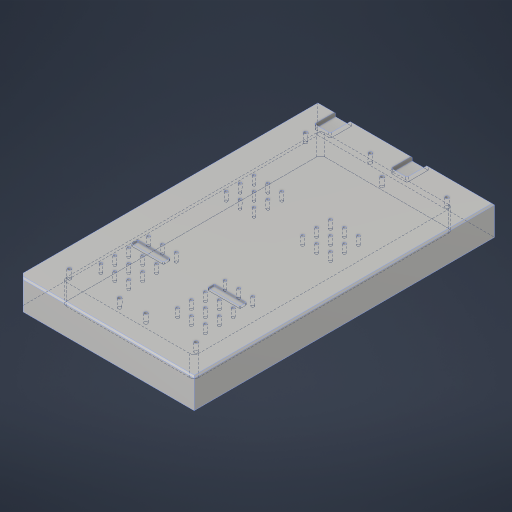
# Autodesk Inventor part: Assembly Plate
Saved by Autodesk Inventor 2024 (Build 280153000, 153)
## iProperties
Created: 2021-01-11
Part Number: Assembly Plate
Material: Aluminum 6061
Document SubType Name: Modeling
Designer: caleb
Density: 2.7 g/cm^3
Appearance: Aluminum - Flat
Author: caleb
Autodesk Inventor part; units mm, degrees
ref_plane "YZ Plane" through (0, 0, 0) normal (1, 0, 0) x (0, 1, 0)
ref_plane "XZ Plane" through (0, 0, 0) normal (0, 1, 0) x (-1, 0, 0)
ref_plane "XY Plane" through (0, 0, 0) normal (0, 0, 1) x (1, 0, 0)
sketch "Sketch1" plane through (0, 0, 0) normal (0, 1, 0) x (-1, 0, 0)
  line L0 (-63.5, 107.95) -> (63.5, 107.95)
  line L1 (63.5, 107.95) -> (63.5, -107.95)
  line L2 (63.5, -107.95) -> (-63.5, -107.95)
  line L3 (-63.5, -107.95) -> (-63.5, 107.95)
  line L4 (-63.5, 107.95) -> (63.5, -107.95) construction
  line L5 (63.5, 107.95) -> (-63.5, -107.95) construction
  point P0 (0, 0)
  dimension "d0" = 127
  dimension "d1" = 215.9
  constraints: 12 end point, 2 midpoint, 2 parallel, 1 horizontal, 1 perpendicular
  measures "d0" distance of L1.end L2.end
  measures "d1" distance of L0.end L1.end
extrude "Extrusion1" add sketch "Sketch1" along normal blind 21.14
sketch "Sketch9" plane through (0, 21.14, 0) normal (0, 1, 0) x (1, 0, 0)
  line L0 (-63.5, 107.95) -> (-63.5, -107.95) projected
  line L1 (-63.5, -107.95) -> (63.5, -107.95) projected
  point P0 (0, 0)
  point P1 (-48.5, -85.65)
  point P2 (-12.4, -85.65)
  point P3 (-48.5, 84.134)
  point P4 (-12.4, 94.65)
  point P5 (42.6, 94.65)
  point P6 (6.5, 84.134)
  point P7 (42.6, -85.65)
  point P8 (6.5, -85.65)
  dimension "d126" = 36.1
  dimension "d127" = 169.784
  dimension "d128" = 180.3
  dimension "d129" = 15
  dimension "d130" = 22.3
  dimension "d164" = 55
  constraints: 2 vertical alignment, 1 horizontal, 1 horizontal alignment, 4 other
  measures "d126" distance of point (-12.4, -85.65) point (-48.5, -85.65)
  measures "d127" distance of point (-48.5, 84.134) point (-48.5, -85.65)
  measures "d128" distance of point (-12.4, 94.65) point (-12.4, -85.65)
  measures "d129" distance from line of L0 point (-48.5, -85.65)
  measures "d130" vertical distance of L0.end point (-48.5, -85.65)
  measures "d164" distance of point (-12.4, 94.65) point (42.6, 94.65)
hole "Hole2" at (-48.5, 21.14, 85.65) at (-12.4, 21.14, 85.65) at (-48.5, 21.14, -84.134) at (-12.4, 21.14, -94.65) at (6.5, 21.14, 85.65) at (42.6, 21.14, 85.65) at (6.5, 21.14, -84.134) at (42.6, 21.14, -94.65) direction (0, -1, 0) diameter 2.5 end through all
sketch "Sketch10" plane through (0, 21.14, 0) normal (0, 1, 0) x (1, 0, 0)
  line L0 (-41.5, -47.65) -> (-19.4, -47.65)
  line L1 (-18.9, -47.15) -> (-18.9, -43.45)
  line L2 (-19.4, -42.95) -> (-41.5, -42.95)
  line L3 (-42, -43.45) -> (-42, -47.15)
  line L4 (-63.5, -107.95) -> (63.5, -107.95) projected
  line L5 (-63.5, 107.95) -> (-63.5, -107.95) projected
  arc A0 (-42, -47.15) -> (-41.5, -47.65) centre (-41.5, -47.15) ccw
  arc A1 (-41.5, -42.95) -> (-42, -43.45) centre (-41.5, -43.45) ccw
  arc A2 (-18.9, -43.45) -> (-19.4, -42.95) centre (-19.4, -43.45) ccw
  arc A3 (-19.4, -47.65) -> (-18.9, -47.15) centre (-19.4, -47.15) ccw
  arc A4 (13.5, -42.95) -> (13, -43.45) centre (13.5, -43.45) ccw
  arc A5 (36.1, -43.45) -> (35.6, -42.95) centre (35.6, -43.45) ccw
  line L6 (13, -43.45) -> (13, -47.15)
  line L7 (36.1, -47.15) -> (36.1, -43.45)
  line L8 (13.5, -47.65) -> (35.6, -47.65)
  arc A6 (13, -47.15) -> (13.5, -47.65) centre (13.5, -47.15) ccw
  arc A7 (35.6, -47.65) -> (36.1, -47.15) centre (35.6, -47.15) ccw
  line L9 (35.6, -42.95) -> (13.5, -42.95)
  point P0 (0, 0)
  point P1 (-42, -47.65)
  point P2 (-18.9, -42.95)
  point P3 (-18.9, -47.65)
  point P4 (-42, -42.95)
  point P5 (13, -47.65)
  point P6 (13, -42.95)
  point P7 (36.1, -42.95)
  point P8 (36.1, -47.65)
  dimension "d140" = 60.3
  dimension "d141" = 65
  dimension "d142" = 21.5
  dimension "d143" = 23.1
  dimension "d144" = 0.5
  dimension "d171" = 55
  constraints: 16 end point, 16 point on circle, 16 point on line, 8 centre point, 8 tangent, 3 equal radius, 2 horizontal, 2 parallel, 1 perpendicular, 24 other
  measures "d140" distance between parallel lines of L4 L0
  measures "d141" distance between parallel lines of L4 L2
  measures "d142" distance between parallel lines of L5 L3
  measures "d143" distance between parallel lines of L1 L3
  measures "d144" radius of A0
  measures "d171" distance of L3.start L6.start
extrude "Extrusion8" cut sketch "Sketch10" against normal blind 1.5
sketch "Sketch11" plane through (0, 21.14, 0) normal (0, 1, 0) x (1, 0, 0)
  line L0 (63.5, 107.95) -> (-63.5, 107.95) projected
  line L1 (-50.7, 107.95) -> (-39.2, 107.95)
  line L2 (-39.2, 107.95) -> (-39.2, 93.65)
  line L3 (-40.2, 92.65) -> (-49.7, 92.65)
  line L4 (-50.7, 93.65) -> (-50.7, 107.95)
  line L5 (-63.5, 107.95) -> (-63.5, -107.95) projected
  arc A0 (-50.7, 93.65) -> (-49.7, 92.65) centre (-49.7, 93.65) ccw
  arc A1 (-40.2, 92.65) -> (-39.2, 93.65) centre (-40.2, 93.65) ccw
  line L6 (4.3, 107.95) -> (15.8, 107.95)
  line L7 (15.8, 107.95) -> (15.8, 93.65)
  line L8 (14.8, 92.65) -> (5.3, 92.65)
  line L9 (4.3, 93.65) -> (4.3, 107.95)
  arc A2 (4.3, 93.65) -> (5.3, 92.65) centre (5.3, 93.65) ccw
  arc A3 (14.8, 92.65) -> (15.8, 93.65) centre (14.8, 93.65) ccw
  point P0 (0, 0)
  point P1 (-39.2, 92.65)
  point P2 (-50.7, 92.65)
  point P3 (-39.2, 100.8)
  point P4 (15.8, 92.65)
  point P5 (4.3, 92.65)
  point P6 (15.8, 100.8)
  dimension "d145" = 12.8
  dimension "d146" = 24.3
  dimension "d147" = 15.3
  dimension "d150" = 1
  dimension "d178" = 55
  constraints: 16 end point, 9 point on line, 8 point on circle, 4 centre point, 4 tangent, 2 horizontal, 2 parallel, 1 equal radius, 1 midpoint, 1 perpendicular, 17 other
  measures "d145" distance between parallel lines of L5 L4
  measures "d146" distance from line of point (-39.2, 100.8) L5
  measures "d147" distance between parallel lines of L0 L3
  measures "d150" radius of A0
  measures "d178" distance of L1.start L6.start
extrude "Extrusion9" cut sketch "Sketch11" against normal blind 3.25
chamfer "Chamfer2" distance 1 angle 45 6 edges at (63.5, 21.14, 0) (-57.1, 21.14, -107.95) (-17.45, 21.14, -107.95) (39.65, 21.14, -107.95) (-63.5, 21.14, 0) (0, 21.14, 107.95)
sketch "Sketch12" plane through (0, 0, 0) normal (0, -1, 0) x (1, 0, 0)
  line L0 (-47.5, -96.95) -> (41.5, -96.95)
  line L1 (44.5, -93.95) -> (44.5, 85.95)
  line L2 (41.5, 88.95) -> (-47.5, 88.95)
  line L3 (-50.5, 85.95) -> (-50.5, -93.95)
  line L4 (63.5, -107.95) -> (63.5, 107.95) projected
  line L5 (63.5, 107.95) -> (-63.5, 107.95) projected
  arc A0 (44.5, 85.95) -> (41.5, 88.95) centre (41.5, 85.95) ccw
  arc A1 (-47.5, 88.95) -> (-50.5, 85.95) centre (-47.5, 85.95) ccw
  arc A2 (-50.5, -93.95) -> (-47.5, -96.95) centre (-47.5, -93.95) ccw
  arc A3 (41.5, -96.95) -> (44.5, -93.95) centre (41.5, -93.95) ccw
  line L6 (-63.5, -107.95) -> (-63.5, 107.95) projected
  line L7 (63.5, -107.95) -> (15.8, -107.95) projected
  point P0 (0, 0)
  point P1 (63.5, 103.95)
  point P2 (59.5, 107.95)
  point P3 (-39.2, -107.95)
  dimension "d151" = 19
  dimension "d152" = 19
  dimension "d153" = 3
  dimension "d160" = 13
  dimension "d161" = 11
  constraints: 8 end point, 8 point on circle, 8 tangent, 4 centre point, 3 equal radius, 2 parallel, 1 horizontal, 1 perpendicular
  measures "d151" distance between parallel lines of L4 L1
  measures "d152" distance between parallel lines of L5 L2
  measures "d153" radius of A0
  measures "d160" distance between parallel lines of L6 L3
  measures "d161" distance between parallel lines of L7 L0
extrude "Extrusion10" cut sketch "Sketch12" against normal blind 15
chamfer "Chamfer4" distance 4 angle 45 1 edges at (-63.5, 10.07, 107.95)
sketch "Sketch13" plane through (0, 21.14, 0) normal (0, 1, 0) x (1, 0, 0)
  line L0 (-63.5, 107.95) -> (-63.5, -103.95) projected
  line L1 (-59.5, -107.95) -> (63.5, -107.95) projected
  point P0 (0, 0)
  point P1 (-40.5, -70.95)
  point P2 (-40.5, -60.95)
  point P3 (-40.5, -50.95)
  point P4 (-30.5, -70.95)
  point P5 (-30.5, -60.95)
  point P6 (-30.5, -50.95)
  point P7 (-20.5, -70.95)
  point P8 (-20.5, -60.95)
  point P9 (-20.5, -50.95)
  point P10 (-20.5, 39.05)
  point P11 (-20.5, 29.05)
  point P12 (-20.5, 19.05)
  point P13 (-30.5, 39.05)
  point P14 (-30.5, 29.05)
  point P15 (-30.5, 19.05)
  point P16 (-40.5, 39.05)
  point P17 (-40.5, 29.05)
  point P18 (-40.5, 19.05)
  point P19 (34.5, -50.95)
  point P20 (34.5, -60.95)
  point P21 (34.5, -70.95)
  point P22 (24.5, -50.95)
  point P23 (24.5, -60.95)
  point P24 (24.5, -70.95)
  point P25 (14.5, -50.95)
  point P26 (14.5, -60.95)
  point P27 (14.5, -70.95)
  point P28 (34.5, 39.05)
  point P29 (34.5, 29.05)
  point P30 (34.5, 19.05)
  point P31 (24.5, 39.05)
  point P32 (24.5, 29.05)
  point P33 (24.5, 19.05)
  point P34 (14.5, 39.05)
  point P35 (14.5, 29.05)
  point P36 (14.5, 19.05)
  point P37 (-40.5, -36.8096)
  point P38 (-30.5, -36.8096)
  point P39 (-20.5, -36.8096)
  point P40 (14.5, -36.8096)
  point P41 (24.5, -36.8096)
  point P42 (34.5, -36.8096)
  dimension "d185" = 10
  dimension "d188" = 10
  dimension "d193" = 90
  dimension "d196" = 55
  dimension "d199" = 23
  dimension "d200" = 37
  constraints: 2 horizontal, 2 vertical, 35 other
  measures "d185" distance of point (-40.5, -70.95) point (-40.5, -60.95)
  measures "d188" distance of point (-40.5, -70.95) point (-30.5, -70.95)
  measures "d193" distance of point (-20.5, -50.95) point (-20.5, 39.05)
  measures "d196" distance of point (-20.5, -50.95) point (34.5, -50.95)
  measures "d199" distance from line of L0 point (-40.5, -70.95)
  measures "d200" distance from line of L1 point (-40.5, -70.95)
hole "Hole3" at (-40.5, 21.14, 70.95) at (-40.5, 21.14, 60.95) at (-40.5, 21.14, 50.95) at (-30.5, 21.14, 70.95) at (-30.5, 21.14, 60.95) at (-30.5, 21.14, 50.95) at (-20.5, 21.14, 70.95) at (-20.5, 21.14, 60.95) at (-20.5, 21.14, 50.95) at (-20.5, 21.14, -39.05) at (-20.5, 21.14, -29.05) at (-20.5, 21.14, -19.05) at (-30.5, 21.14, -39.05) at (-30.5, 21.14, -29.05) at (-30.5, 21.14, -19.05) at (-40.5, 21.14, -39.05) at (-40.5, 21.14, -29.05) at (-40.5, 21.14, -19.05) at (34.5, 21.14, 50.95) at (34.5, 21.14, 60.95) at (34.5, 21.14, 70.95) at (24.5, 21.14, 50.95) at (24.5, 21.14, 60.95) at (24.5, 21.14, 70.95) at (14.5, 21.14, 50.95) at (14.5, 21.14, 60.95) at (14.5, 21.14, 70.95) at (34.5, 21.14, -39.05) at (34.5, 21.14, -29.05) at (34.5, 21.14, -19.05) at (24.5, 21.14, -39.05) at (24.5, 21.14, -29.05) at (24.5, 21.14, -19.05) at (14.5, 21.14, -39.05) at (14.5, 21.14, -29.05) at (14.5, 21.14, -19.05) at (34.5, 21.14, 36.8096) at (24.5, 21.14, 36.8096) at (14.5, 21.14, 36.8096) at (-20.5, 21.14, 36.8096) at (-30.5, 21.14, 36.8096) at (-40.5, 21.14, 36.8096) direction (0, -1, 0) diameter 2 end through all
body "Solid1"
